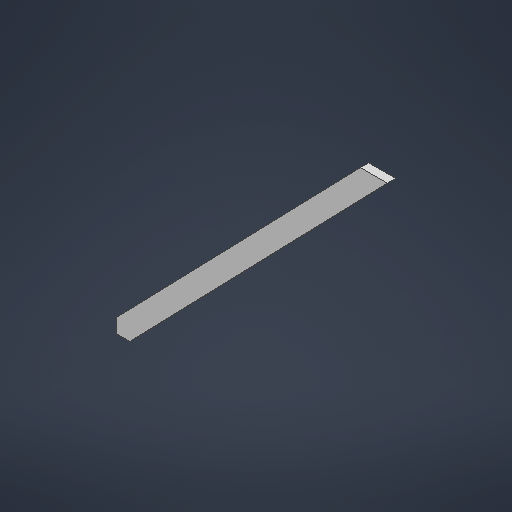
# Autodesk Inventor part: S_2x4x68.525
Saved by Autodesk Inventor 2026 (Build 300175000, 175)
## iProperties
Created: 2025-09-04
Part Number: S_2x4x68.525
Material: Generic
Document SubType Name: Modeling
Designer: trott
Density: 1 g/cm^3
Appearance: Default
Author: trott
Autodesk Inventor part; units mm, degrees
ref_plane "YZ Plane" through (0, 0, 0) normal (1, 0, 0) x (0, 1, 0)
ref_plane "XZ Plane" through (0, 0, 0) normal (0, 1, 0) x (-1, 0, 0)
ref_plane "XY Plane" through (0, 0, 0) normal (0, 0, 1) x (1, 0, 0)
sketch "Sketch1" plane through (0, 0, 0) normal (0, 0, 1) x (1, 0, 0)
  line L0 (-1181.1, -609.6) -> (1181.1, -609.6)
  line L1 (1181.1, -609.6) -> (1181.1, 609.6)
  line L2 (1181.1, 609.6) -> (-1181.1, 609.6)
  line L3 (-1181.1, 609.6) -> (-1181.1, -609.6)
  line L4 (-1181.1, -609.6) -> (1181.1, 609.6) construction
  line L5 (1181.1, -609.6) -> (-1181.1, 609.6) construction
  line L6 (0, 609.6) -> (0, -609.6)
  line L7 (0, 609.6) -> (1181.1, -609.6)
  line L8 (-31.9258, 578.6719) -> (31.9258, 640.5281)
  line L9 (1149.1742, -640.5281) -> (1213.0258, -578.6719)
  line L10 (-31.9258, 578.6719) -> (1149.1742, -640.5281)
  line L11 (1213.0258, -578.6719) -> (31.9258, 640.5281)
  line L12 (-31.9258, 578.6719) -> (-61.8874, 609.6)
  line L13 (1181.1, -609.6) -> (-1181.1, 609.6) construction
  line L14 (0, 609.6) -> (-1181.1, -609.6)
  line L15 (31.9258, 578.6719) -> (-31.9258, 640.5281)
  line L16 (-1149.1742, -640.5281) -> (-1213.0258, -578.6719)
  line L17 (31.9258, 578.6719) -> (-1149.1742, -640.5281)
  line L18 (-1213.0258, -578.6719) -> (-31.9258, 640.5281)
  line L19 (31.9258, 578.6719) -> (61.8874, 609.6)
  point P0 (0, 0)
  point P1 (-1181.1, -545.7163)
  point P2 (-1119.2126, -609.6)
  point P3 (61.8874, 609.6)
  dimension "d0" = 2362.2
  dimension "d1" = 1219.2
  dimension "d3" = 88.9
  dimension "d4" = 88.9
  constraints: 40 end point, 8 symmetric about line, 6 midpoint, 4 perpendicular, 3 point on line, 2 parallel, 1 horizontal
  measures "d0" distance of L2.end L1.end
  measures "d1" distance of L0.end L1.end
  measures "d3" distance of L8.start L8.end
  measures "d4" distance of L9.start L9.end
extrude "Extrusion1" add sketch "Sketch1" along normal blind 38.1 contours L14 L10 L17 L0 | L3 L18 L12 L10 L14 | L14 L6 L10 | L10 L8 L14 | L6 L7 L17 | L2 L8 L12 | L15 L17 L7 | L2 L19 L15
body "Solid1"
